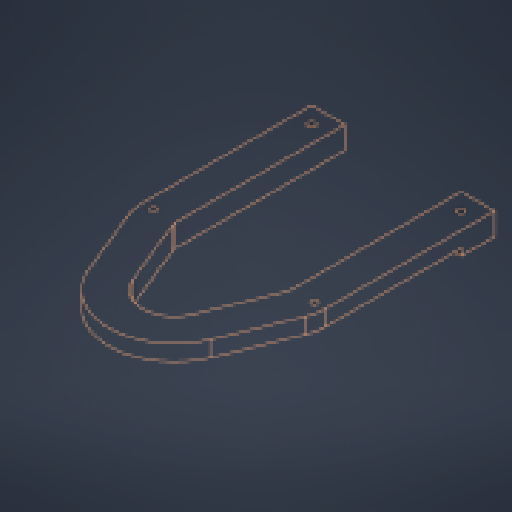
# Autodesk Inventor part: Rear Cover Bracket
Saved by Autodesk Inventor 2023.1 (Build 271208000, 208)
## iProperties
Created: 2023-02-24
Part Number: Rear Cover Bracket
Material: ABS Plastic
Document SubType Name: Modeling
Designer: remop
Density: 1.06 g/cm^3
Appearance: Smooth - Light Orange
Author: remop
Autodesk Inventor part; units mm, degrees
ref_plane "YZ Plane" through (0, 0, 0) normal (1, 0, 0) x (0, 1, 0)
ref_plane "XZ Plane" through (0, 0, 0) normal (0, 1, 0) x (-1, 0, 0)
ref_plane "XY Plane" through (0, 0, 0) normal (0, 0, 1) x (1, 0, 0)
sketch "Sketch13" plane through (0, 0, 0) normal (0, 0, 1) x (1, 0, 0)
  line L0 (-247.6922, -121.6988) -> (-240.7003, -114.707) projected
  line L1 (-240.7003, -114.707) -> (-206.5582, -114.707) projected
  line L2 (-206.5582, -114.707) -> (-199.5663, -121.6988) projected
  line L3 (-199.5663, -121.6988) -> (-199.5663, -165.5825) projected
  arc A0 (-199.7872, -166.7122) -> (-199.5663, -165.5825) centre (-202.5663, -165.5825) ccw projected
  line L4 (-199.7872, -166.7122) -> (-212.0494, -196.8785) projected
  arc A1 (-235.2091, -196.8785) -> (-212.0494, -196.8785) centre (-223.6293, -192.1714) ccw projected
  line L5 (-235.2091, -196.8785) -> (-247.4714, -166.7122) projected
  arc A2 (-247.6922, -165.5825) -> (-247.4714, -166.7122) centre (-244.6922, -165.5825) ccw projected
  line L6 (-247.6922, -165.5825) -> (-247.6922, -121.6988) projected
  circle A3 centre (-238.6293, -136.1714) radius 4 projected
  circle A4 centre (-238.6293, -166.1714) radius 4 projected
  circle A5 centre (-208.6293, -166.1714) radius 4 projected
  circle A6 centre (-208.6293, -136.1714) radius 4 projected
  circle A7 centre (-223.6293, -151.1714) radius 13 projected
  line L7 (26.8154, -89.707) -> (-473.1846, -89.707) projected
  line L8 (26.8154, -104.707) -> (-473.1846, -104.707) projected
  line L9 (-197.5663, -165.5825) -> (-197.5663, -120.8704)
  line L10 (-197.5663, -120.8704) -> (-205.7298, -112.707)
  line L11 (-205.7298, -112.707) -> (-241.5288, -112.707)
  line L12 (-241.5288, -112.707) -> (-249.6922, -120.8704)
  line L13 (-249.6922, -120.8704) -> (-249.6922, -165.5825)
  arc A8 (-249.6922, -165.5825) -> (-249.3242, -167.4653) centre (-244.6922, -165.5825) ccw
  line L14 (-249.3242, -167.4653) -> (-237.0619, -197.6316)
  arc A9 (-237.0619, -197.6316) -> (-210.1966, -197.6316) centre (-223.6293, -192.1714) ccw
  line L15 (-210.1966, -197.6316) -> (-197.9344, -167.4653)
  arc A10 (-197.9344, -167.4653) -> (-197.5663, -165.5825) centre (-202.5663, -165.5825) ccw
  line L16 (-182.5663, -165.5825) -> (-182.5663, -114.6572)
  line L17 (-182.5663, -114.6572) -> (-199.5166, -97.707)
  line L18 (-199.5166, -97.707) -> (-247.742, -97.707)
  line L19 (-247.742, -97.707) -> (-264.6922, -114.6572)
  line L20 (-264.6922, -114.6572) -> (-264.6922, -165.5825)
  arc A11 (-264.6922, -165.5825) -> (-263.22, -173.1138) centre (-244.6922, -165.5825) ccw
  line L21 (-263.22, -173.1138) -> (-250.9578, -203.2801)
  arc A12 (-250.9578, -203.2801) -> (-196.3008, -203.2801) centre (-223.6293, -192.1714) ccw
  line L22 (-196.3008, -203.2801) -> (-184.0385, -173.1138)
  arc A13 (-184.0385, -173.1138) -> (-182.5663, -165.5825) centre (-202.5663, -165.5825) ccw
  line L23 (-182.5663, -114.6572) -> (-182.5663, -89.707)
  line L24 (-264.6922, -114.6572) -> (-264.6922, -89.707)
  line L25 (-197.5663, -120.8704) -> (-197.5663, -89.707)
  line L26 (-249.6922, -120.8704) -> (-249.6922, -89.707)
  line L27 (-218.4828, -188.996) -> (-218.1293, -188.6424) projected
  line L28 (-218.1293, -188.6424) -> (-218.1293, -185.996) projected
  line L29 (-218.1293, -185.996) -> (-229.1293, -185.996) projected
  line L30 (-229.1293, -185.996) -> (-229.1293, -188.6424) projected
  line L31 (-229.1293, -188.6424) -> (-228.7757, -188.996) projected
  line L32 (-228.7757, -188.996) -> (-218.4828, -188.996) projected
  line L33 (-228.9525, -189.3022) -> (-229.4355, -189.1728) projected
  line L34 (-229.4355, -189.1728) -> (-231.7273, -190.496) projected
  line L35 (-231.7273, -190.496) -> (-226.2273, -200.0223) projected
  line L36 (-226.2273, -200.0223) -> (-223.9355, -198.6991) projected
  line L37 (-223.9355, -198.6991) -> (-223.806, -198.2161) projected
  line L38 (-223.806, -198.2161) -> (-228.9525, -189.3022) projected
  line L39 (-223.4525, -198.2161) -> (-223.3231, -198.6991) projected
  line L40 (-223.3231, -198.6991) -> (-221.0312, -200.0223) projected
  line L41 (-221.0312, -200.0223) -> (-215.5312, -190.496) projected
  line L42 (-215.5312, -190.496) -> (-217.8231, -189.1728) projected
  line L43 (-217.8231, -189.1728) -> (-218.306, -189.3022) projected
  line L44 (-218.306, -189.3022) -> (-223.4525, -198.2161) projected
  point P0 (0, 0)
  dimension "d26" = 2
  dimension "d27" = 15
  constraints: 36 end point, 12 point on circle, 6 centre point, 4 perpendicular, 4 point on line, 18 other
  measures "d26" distance between parallel lines of L9 L3
  measures "d27" distance between parallel lines of L16 L9
extrude "Extrusion14" add sketch "Sketch13" along normal blind 10 contours L23 L8 L17 L25 L7 | L23 L17 L8 | L26 L19 L8 L24 L7 | L17 L8 L25 | L17 L16 A13 L22 A12 L21 A11 L20 L19 L8 L26 L13 A8 L14 A9 L15 A10 L9 L25 | L26 L8 L19 | L8 L19 L24
sketch "Sketch14" plane through (0, 0, 0) normal (0, 0, -1) x (-1, 0, 0)
  line L0 (249.6922, -165.5825) -> (249.6922, -89.707) projected
  arc A0 (249.3242, -167.4653) -> (249.6922, -165.5825) centre (244.6922, -165.5825) ccw projected
  line L1 (237.0619, -197.6316) -> (249.3242, -167.4653) projected
  arc A1 (210.1966, -197.6316) -> (237.0619, -197.6316) centre (223.6293, -192.1714) ccw projected
  line L2 (197.9344, -167.4653) -> (210.1966, -197.6316) projected
  arc A2 (197.5663, -165.5825) -> (197.9344, -167.4653) centre (202.5663, -165.5825) ccw projected
  line L3 (197.5663, -89.707) -> (197.5663, -165.5825) projected
  line L4 (182.5663, -89.707) -> (197.5663, -89.707) projected
  line L5 (182.5663, -165.5825) -> (182.5663, -89.707) projected
  arc A3 (182.5663, -165.5825) -> (184.0385, -173.1138) centre (202.5663, -165.5825) ccw projected
  line L6 (196.3008, -203.2801) -> (184.0385, -173.1138) projected
  arc A4 (196.3008, -203.2801) -> (250.9578, -203.2801) centre (223.6293, -192.1714) ccw projected
  line L7 (263.22, -173.1138) -> (250.9578, -203.2801) projected
  arc A5 (263.22, -173.1138) -> (264.6922, -165.5825) centre (244.6922, -165.5825) ccw projected
  line L8 (264.6922, -89.707) -> (264.6922, -165.5825) projected
  line L9 (249.6922, -89.707) -> (264.6922, -89.707) projected
  line L10 (185.5663, -92.707) -> (194.5663, -92.707)
  line L11 (194.5663, -92.707) -> (194.5663, -165.5825)
  arc A6 (194.5663, -165.5825) -> (195.1552, -168.595) centre (202.5663, -165.5825) ccw
  line L12 (195.1552, -168.595) -> (207.4175, -198.7613)
  arc A7 (207.4175, -198.7613) -> (239.8411, -198.7613) centre (223.6293, -192.1714) ccw
  line L13 (239.8411, -198.7613) -> (252.1033, -168.595)
  arc A8 (252.1033, -168.595) -> (252.6922, -165.5825) centre (244.6922, -165.5825) ccw
  line L14 (252.6922, -165.5825) -> (252.6922, -92.707)
  line L15 (252.6922, -92.707) -> (261.6922, -92.707)
  line L16 (261.6922, -92.707) -> (261.6922, -165.5825)
  arc A9 (260.4408, -171.9841) -> (261.6922, -165.5825) centre (244.6922, -165.5825) ccw
  line L17 (260.4408, -171.9841) -> (248.1786, -202.1504)
  arc A10 (199.0799, -202.1504) -> (248.1786, -202.1504) centre (223.6293, -192.1714) ccw
  line L18 (199.0799, -202.1504) -> (186.8177, -171.9841)
  arc A11 (185.5663, -165.5825) -> (186.8177, -171.9841) centre (202.5663, -165.5825) ccw
  line L19 (185.5663, -165.5825) -> (185.5663, -92.707)
  line L20 (194.5663, -92.707) -> (194.5663, -89.707)
  line L21 (182.5663, -89.707) -> (197.5663, -89.707) projected
  line L22 (252.6922, -92.707) -> (252.6922, -89.707)
  line L23 (197.5663, -89.707) -> (197.5663, -165.5825) projected
  line L24 (197.5663, -104.707) -> (182.5663, -104.707)
  line L25 (264.6922, -89.707) -> (264.6922, -165.5825) projected
  line L26 (264.6922, -104.707) -> (249.6922, -104.707)
  point P0 (0, 0)
  point P1 (194.5663, -104.707)
  point P2 (252.6922, -104.707)
  dimension "d33" = 3
  dimension "d34" = 15
  constraints: 28 end point, 12 point on circle, 6 centre point, 6 point on line, 3 perpendicular, 1 horizontal alignment, 1 vertical, 15 other
  measures "d33" distance between parallel lines of L3 L11
  measures "d34" distance between parallel lines of L9 L26
extrude "Extrusion15" cut sketch "Sketch14" against normal blind 3 contours L26 L16 A9 L17 A10 L18 A11 L19 L24 L11 A6 L12 A7 L13 A8 L14 | L26 L8 A5 L7 A4 L6 A3 L5 L24 L19 A11 L18 A10 L17 A9 L16
sketch "Sketch15" plane through (0, 0, 3) normal (0, 0, -1) x (-1, 0, 0)
  line L0 (182.5663, -165.5825) -> (182.5663, -104.707) projected
  line L1 (264.6922, -104.707) -> (264.6922, -165.5825) projected
  point P0 (0, 0)
  point P1 (187.5663, -165.5825)
  point P2 (259.6922, -165.5825)
  dimension "d35" = 5
  dimension "d36" = 5
  constraints: 2 horizontal alignment
  measures "d35" distance from line of L0 point (187.566, -165.582)
  measures "d36" distance from line of L1 point (259.692, -165.582)
hole "Hole1" at (-187.5663, -165.5825, 3) at (-259.6922, -165.5825, 3) direction (0, 0, 1) diameter 2.9 end through all
sketch "Sketch16" plane through (0, 0, 10) normal (0, 0, 1) x (1, 0, 0)
  line L0 (-264.6922, -89.707) -> (-264.6922, -165.5825) projected
  line L1 (-182.5663, -165.5825) -> (-182.5663, -89.707) projected
  point P0 (0, 0)
  point P1 (-257.1922, -97.207)
  point P2 (-190.0663, -97.207)
  dimension "d44" = 7.5
  dimension "d45" = 7.5
  dimension "d46" = 7.5
  constraints: 1 horizontal alignment
  measures "d44" horizontal distance of L0.start point (-257.192, -97.207)
  measures "d45" distance from line of L1 point (-190.066, -97.207)
  measures "d46" distance from line of L0 point (-257.192, -97.207)
hole "Hole2" at (-257.1922, -97.207, 10) at (-190.0663, -97.207, 10) direction (0, 0, -1) diameter 3.2 end through all
equation "\"d36\" = d35"
equation "\"d45\" = d44"
equation "\"d46\" = d44"
body "Solid11"
